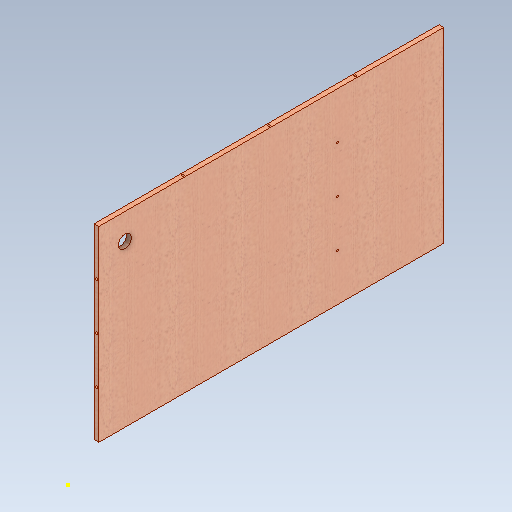
# Autodesk Inventor part: FondoMuralla
Saved by Autodesk Inventor 2020.3 (Build 243373000, 373)
## iProperties
Created: 2020-10-27
Part Number: FondoMuralla
Material: Madera (roble)
Document SubType Name: Modeling
Designer: codig
Density: 0.76 g/cm^3
Appearance: Roble blanco - Natural brillo medio
Mass: 17195 g
Surface Area: 19939.6 cm^2
Volume: 17195 cm^3
Author: codig
Autodesk Inventor part; units mm, degrees
ref_plane "YZ Plane" through (0, 0, 0) normal (1, 0, 0) x (0, 1, 0)
ref_plane "XZ Plane" through (0, 0, 0) normal (0, 1, 0) x (-1, 0, 0)
ref_plane "XY Plane" through (0, 0, 0) normal (0, 0, 1) x (1, 0, 0)
sketch "Boceto1" plane through (0, 0, 0) normal (1, 0, 0) x (0, 1, 0)
  line L0 (100, -100) -> (820, -100)
  line L1 (820, -100) -> (820, -1428)
  line L2 (820, -1428) -> (100, -1428)
  line L3 (100, -1428) -> (100, -100)
  point P0 (0, 0)
  constraints: 8 end point, 2 parallel, 1 horizontal, 1 perpendicular
extrude "Extrusión1" add sketch "Boceto1" along normal blind 18
sketch "Boceto2" plane through (0, 0, 0) normal (-1, 0, 0) x (0, 0, 1)
  point P0 (0, 0)
sketch "Boceto3" plane through (0, 820, -100) normal (0, 1, 0) x (1, 0, 0)
  line L0 (0, 1328) -> (0, 0) projected
  line L1 (0, 1328) -> (18, 1328) projected
  circle A0 centre (9, 996) radius 4
  circle A1 centre (9, 664) radius 4
  circle A2 centre (9, 332) radius 4
  point P0 (0, -100)
  constraints: 3 centre point
hole "Agujero1" at (9, 820, -1096) at (9, 820, -764) at (9, 820, -432) direction (0, -1, 0) diameter 8 depth 35
sketch "Boceto4" plane through (0, 100, -100) normal (0, 0, 1) x (1, 0, 0)
  circle A0 centre (9, 180) radius 4
  circle A1 centre (9, 360) radius 4
  circle A2 centre (9, 540) radius 4
  line L0 (0, 720) -> (18, 720) projected
  point P0 (0, -100)
  constraints: 3 centre point
hole "Agujero2" at (9, 640, -100) at (9, 460, -100) at (9, 280, -100) direction (0, 0, -1) diameter 8 depth 35
sketch "Boceto5" plane through (0, 100, -1428) normal (0, 0, -1) x (-1, 0, 0)
  circle A0 centre (-9, 540) radius 4
  circle A1 centre (-9, 360) radius 4 projected
  circle A2 centre (-9, 360) radius 4
  circle A3 centre (-9, 180) radius 4 projected
  circle A4 centre (-9, 180) radius 4
  point P0 (0, -100)
  constraints: 3 centre point, 2 coincident
hole "Agujero3" at (9, 280, -1428) at (9, 460, -1428) at (9, 640, -1428) direction (0, 0, 1) diameter 8 depth 35
sketch "Boceto6" plane through (18, 0, 0) normal (1, 0, 0) x (0, 0, -1)
  line L0 (100, 100) -> (1428, 100) projected
  circle A0 centre (1019, 640) radius 4
  circle A1 centre (1019, 460) radius 4
  circle A2 centre (1019, 280) radius 4
  point P0 (0, 0)
  constraints: 3 centre point
hole "Agujero4" at (18, 280, -1019) at (18, 460, -1019) at (18, 640, -1019) direction (-1, 0, 0) diameter 8 depth 10
sketch "Boceto7" plane through (0, 100, -1428) normal (0, -1, 0) x (1, 0, 0)
  circle A0 centre (9, 332) radius 4 projected
  circle A1 centre (9, 332) radius 4
  circle A2 centre (9, 664) radius 4 projected
  circle A3 centre (9, 664) radius 4
  circle A4 centre (9, 996) radius 4 projected
  circle A5 centre (9, 996) radius 4
  point P0 (0, 1428)
  constraints: 3 centre point, 3 coincident
hole "Agujero5" at (9, 100, -1096) at (9, 100, -764) at (9, 100, -432) direction (0, 1, 0) diameter 8 depth 23
sketch "Boceto8" plane through (18, 0, 0) normal (1, 0, 0) x (0, 0, -1)
  circle A0 centre (200, 720) radius 25
  point P0 (0, 0)
  constraints: 1 centre point
hole "Agujero6" at (18, 720, -200) direction (-1, 0, 0) diameter 50 end through all
